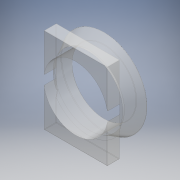
# Autodesk Inventor part: Painel FMC v4 anel de silicone Branco
Saved by Autodesk Inventor 2016 (Build 200138000, 138)
## iProperties
Created: 2010-08-30
Part Number: Painel FMC v4 anel de silicone Branco
Material: ABS Plastic
Document SubType Name: Modeling
Designer: fernando.santanna
Density: 1.06 g/cm^3
Appearance: Smooth - White
Sending System: Autodesk Inventor 2010
Preprocessor: Autodesk Inventor 2010
Title: C:\Documents and Settings\mtravers\Desktop\XFM85-0001.stp
Author: mtravers
Autodesk Inventor part; units mm, degrees
ref_plane "Work Plane13" through (159.7554, 142.178, 12.7) normal (0, 1, 0) x (1, 0, 0)
sketch "Sketch2" plane through (159.7554, 142.178, 12.7) normal (0, 1, 0) x (1, 0, 0)
  circle A0 centre (4.06, 5.55) radius 4.25
  dimension "d11" = 8.5
  constraints: 1 centre point
  measures "d11" diameter of A0
extrude "Extrusion2" [suppressed]
ref_plane "Work Plane11" through (159.7554, 139.678, 0) normal (0, -1, 0) x (1, 0, 0)
sketch "Sketch6" plane through (159.7554, 139.678, 0) normal (0, -1, 0) x (1, 0, 0)
  arc A0 (0.2, 5.3715) -> (0.2, 8.9285) centre (4.06, 7.15) ccw projected
  line L0 (0.2, 8.9285) -> (0.2, 11.75) projected
  line L1 (0.2, 12.4) -> (7.92, 12.4)
  line L2 (7.92, 12.4) -> (7.92, 1.9)
  line L3 (7.92, 1.9) -> (0.2, 1.9)
  line L4 (0.2, 1.9) -> (0.2, 12.4)
  dimension "d47" = 1
  dimension "d48" = 1
  dimension "d49" = 10.5
  dimension "d50" = 7.72
  dimension "d53" = 3.86
  constraints: 8 end point, 2 parallel, 1 horizontal, 1 perpendicular, 1 point on line
  measures "d47" distance edge to line of A0 L1
  measures "d48" distance edge to line of A0 L3
  measures "d49" distance of L1.end L2.end
  measures "d50" distance of L2.end L3.end
  measures "d53" distance from line of L4 A0.centre
extrude "Extrusion6" add sketch "Sketch6" along normal blind 1 contours L4 A0 L2 | A0 L2 L3 L4 | L0 L4 L1 L2 A0
ref_plane "Work Plane8" through (159.7554, 139.678, 0) normal (0, 1, 0) x (1, 0, 0)
sketch "Sketch7" plane through (159.7554, 139.678, 0) normal (0, 1, 0) x (1, 0, 0)
  circle A0 centre (4.06, -7.15) radius 4.25 projected
  line L0 (0.2, -1.9) -> (0.2, -12.4) projected
  line L1 (7.92, -12.4) -> (7.92, -1.9) projected
  line L2 (0.2, -1.9) -> (0.2, -12.4) projected
  line L3 (7.92, -12.4) -> (7.92, -1.9) projected
  line L4 (0.2, -12.4) -> (7.92, -12.4) projected
  line L5 (7.92, -1.9) -> (0.2, -1.9) projected
  line L6 (0.2, -12.4) -> (7.92, -12.4) projected
  line L7 (7.92, -1.9) -> (0.2, -1.9) projected
  point P0 (-159.7554, 0)
extrude "Extrusion7" add sketch "Sketch7" along normal blind 0.5 contours L1 A0 L0 | A0 L0 L5 L1 | L1 L4 L0 A0
sketch "Sketch8" plane through (159.7554, 140.178, 0) normal (0, 1, 0) x (1, 0, 0)
  line L0 (0.2, -1.9) -> (0.2, -12.4) projected
  line L1 (7.92, -12.4) -> (7.92, -1.9) projected
  circle A0 centre (4.06, -7.15) radius 5.4047 projected
  arc A1 (7.92, -8.9285) -> (7.92, -5.3715) centre (4.06, -7.15) ccw projected
  arc A2 (0.2, -8.9285) -> (7.92, -8.9285) centre (4.06, -7.15) ccw projected
  arc A3 (0.2, -5.3715) -> (0.2, -8.9285) centre (4.06, -7.15) ccw projected
  arc A4 (7.92, -5.3715) -> (0.2, -5.3715) centre (4.06, -7.15) ccw projected
  circle A5 centre (4.06, -7.15) radius 5.4047 projected
  line L2 (0.2, -12.4) -> (7.92, -12.4) projected
  line L3 (7.92, -1.9) -> (0.2, -1.9) projected
  point P0 (-159.7554, 0)
  constraints: 1 other
extrude "Extrusion8" add sketch "Sketch8" along normal blind 0.2 contours A4 L1 A2 L0 | L0 A3 | A1 L1
ref_plane "Work Plane2" through (163.8154, 140.378, 7.15) normal (0, 0, 1) x (0, 1, 0)
sketch "Sketch11" plane through (163.8154, 140.378, 7.15) normal (0, 0, 1) x (0, 1, 0)
  line L0 (-168.8135, 0) -> (30.2356, 0) projected
  line L1 (0, -4.25) -> (0, 4.25) projected
  line L2 (1.8, -5.4047) -> (1.8, 5.4047) projected
  line L3 (1.8, -5.4047) -> (-0.2, -4.25) projected
  line L4 (1.8, 0) -> (1.8, -5.4047)
  line L5 (0, -4.3655) -> (0, 0)
  line L6 (0, 0) -> (1.8, 0)
  line L7 (1.8, -5.4047) -> (0, -4.3655)
  line L8 (0, -4.25) -> (1.8, -5.2892)
  point P0 (-140.378, 163.8154)
  dimension "d60" = 0.1
  constraints: 10 end point, 3 collinear, 3 point on line, 2 midpoint, 1 parallel
  measures "d60" distance between parallel lines of L3 L8
revolve "Revolution1" add sketch "Sketch11" angle 360 about axis through (163.8154, 140.378, 7.15) along (0, 1, 0) contours L0 L2 L8 L1
sketch "Sketch12" plane through (163.8154, 142.178, 7.15) normal (0, 1, 0) x (1, 0, 0)
  circle A0 centre (0, 0) radius 3.9
  point P0 (-163.8154, 7.15)
  dimension "d62" = 7.8
  constraints: 1 centre point
  measures "d62" diameter of A0
extrude "Extrusion9" cut sketch "Sketch12" against normal through all
fillet "Fillet1" radius 0.5 1 edges at (163.8154, 140.178, 2.9)
fillet "Fillet2" radius 0.05 22 edges at (167.6754, 139.428, 1.9) (163.8154, 140.178, 1.9) (167.6754, 140.23, 4.9804) (167.6754, 140.178, 3.2286) (167.6754, 138.678, 4.2464) (163.8154, 138.678, 1.9) (159.9554, 139.428, 1.9) (159.9554, 140.23, 4.9804) (159.9554, 140.178, 3.2286) (159.9554, 138.678, 4.2464) (159.9554, 138.678, 10.0536) (159.9554, 140.178, 10.6642) (159.9554, 139.428, 12.4) (163.8154, 140.178, 12.4) (163.8154, 138.678, 12.4) (167.6754, 139.428, 12.4) (167.6754, 140.178, 10.6642) (167.6754, 138.678, 10.0536) (168.7344, 142.178, 5.2058) (161.8713, 142.178, 12.069) (163.8154, 142.178, 1.8608) (159.9154, 142.178, 7.15)
equation "\"d50\" = 2 * d53"
body "Solid2"
